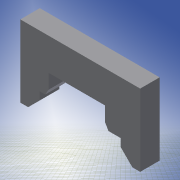
# Autodesk Inventor part: _WT_Aufnahme_Antriebseinheit4
Saved by Autodesk Inventor 2019 (Build 230136000, 136)
## iProperties
Created: 2025-05-01
Part Number: _WT_Aufnahme_Antriebseinheit4
Material: Generisch
Document SubType Name: Modeling
Designer: RP
Density: 1 g/cm^3
Appearance: Vorgabe
Author: RP
Autodesk Inventor part; units mm, degrees
ref_plane "YZ Plane" through (0, 0, 0) normal (1, 0, 0) x (0, 1, 0)
ref_plane "XZ Plane" through (0, 0, 0) normal (0, 1, 0) x (-1, 0, 0)
ref_plane "XY Plane" through (0, 0, 0) normal (0, 0, 1) x (1, 0, 0)
sketch "Skizze1" plane through (0, 0, 0) normal (0, 0, 1) x (1, 0, 0)
  line L0 (-19, -14.5) -> (-19, -10.5)
  line L1 (-19, -10.5) -> (-16.2321, -10.5)
  line L2 (-16.2321, -10.5) -> (-14.5, -7.5)
  line L3 (-14.5, -7.5) -> (-14.5, 0)
  line L4 (-14.5, 0) -> (14.5, 0)
  line L5 (14.5, 0) -> (14.5, -7.5)
  line L6 (14.5, -7.5) -> (16.2321, -10.5)
  line L7 (16.2321, -10.5) -> (22.5, -10.5)
  line L8 (22.5, -10.5) -> (22.5, -14.5)
  line L9 (22.5, -14.5) -> (28.5, -20.5)
  line L10 (28.5, -20.5) -> (32.5, -20.5)
  line L11 (32.5, -20.5) -> (32.5, 16.5)
  line L12 (32.5, 16.5) -> (-29, 16.5)
  line L13 (-29, 16.5) -> (-29, -20.5)
  line L14 (-29, -20.5) -> (-25, -20.5)
  line L15 (-25, -20.5) -> (-19, -14.5)
  line L16 (0, 0) -> (0, -29.3821)
  dimension "d5" = 29
  dimension "d6" = 16.5
  dimension "d7" = 7.5
  dimension "d8" = 4.5
  dimension "d10" = 41.5
  dimension "d12" = 30
  dimension "d13" = 10
  dimension "d14" = 10
  dimension "d15" = 10.5
  dimension "d16" = 45
  dimension "d17" = 10
  dimension "d18" = 4
  constraints: 35 end point, 9 perpendicular, 3 parallel, 2 point on line, 2 vertical, 1 collinear, 1 midpoint, 2 other
  measures "d5" distance of L3.end L4.end
  measures "d6" distance between parallel lines of L12 L4
  measures "d7" distance of L2.end L3.end
  measures "d8" distance between parallel lines of L3 L0
  measures "d10" distance between parallel lines of L0 L8
  measures "d12" angle of L2 L3
  measures "d13" distance between parallel lines of L0 L13
  measures "d14" distance between parallel lines of L11 L8
  measures "d15" distance between parallel lines of L1 L4
  measures "d16" angle of L0 L15
  measures "d17" distance between parallel lines of L1 L14
  measures "d18" distance of L0.start L0.end
extrude "Extrusion1" add sketch "Skizze1" along normal mid plane 10
chamfer "Fase1" distance 1 angle 45 2 edges at (-19, -12.5, -5) (-22, -17.5, -5)
